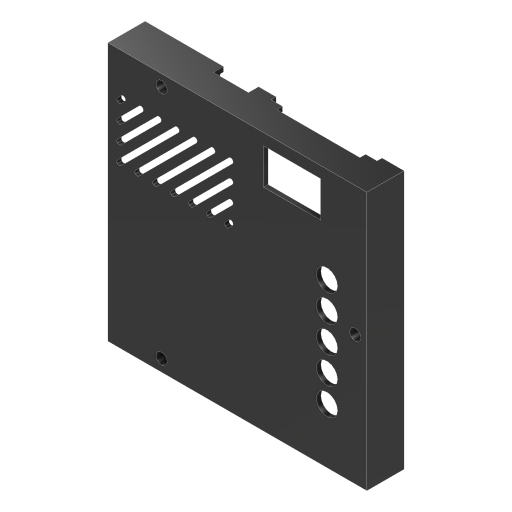
# Autodesk Inventor part: display_cover_part1_back
Saved by Autodesk Inventor 2023 (Build 270158000, 158)
## iProperties
Created: 2024-12-14
Part Number: display_cover_part1_back
Material: Všeobecné
Document SubType Name: Modeling
Designer: Marek
Density: 1 g/cm^3
Appearance: Lesklá – černá
Author: Marek
## iProperties of the stored document display_cover_part1_back_3D tisk.ipt
Created: 2025-02-02
Part Number: display_cover_part1_back_3D tisk
Material: Všeobecné
Document SubType Name: Modeling
Designer: Marek
Density: 1 g/cm^3
Appearance: Výchozí
Author: Marek
Autodesk Inventor part; units mm, degrees
ref_plane "YZ Plane" through (0, 0, 0) normal (1, 0, 0) x (0, 1, 0)
ref_plane "XZ Plane" through (0, 0, 0) normal (0, 1, 0) x (-1, 0, 0)
ref_plane "XY Plane" through (0, 0, 0) normal (0, 0, 1) x (1, 0, 0)
sketch "Náčrt1" plane through (0, 0, 0) normal (0, 0, 1) x (1, 0, 0)
  line L0 (0, 110.95) -> (0, -110.95) projected
  line L1 (-107, 0) -> (115.25, 0) projected
  line L2 (-75.25, 79.25) -> (83.5, 79.25)
  line L3 (83.5, 79.25) -> (83.5, -79.25)
  line L4 (83.5, -79.25) -> (-75.25, -79.25)
  line L5 (-75.25, -79.25) -> (-75.25, 79.25)
  point P0 (0, 0)
  dimension "d0" = 158.75
  dimension "d1" = 158.5
  dimension "d7" = 83.5
  constraints: 8 end point, 2 parallel, 1 horizontal, 1 perpendicular, 1 other
  measures "d0" distance of L3.end L4.end
  measures "d1" distance of L2.end L3.end
  measures "d7" distance between parallel lines of L0 L3
extrude "Vysunutí1" add sketch "Náčrt1" along normal blind 2.8
sketch "Náčrt2" plane through (0, 0, 0) normal (0, 0, -1) x (-1, 0, 0)
  line L0 (75.25, -79.25) -> (-83.5, -79.25) projected
  line L1 (75.25, 79.25) -> (75.25, -79.25) projected
  line L2 (-83.5, 79.25) -> (75.25, 79.25) projected
  line L3 (-83.5, -79.25) -> (-83.5, 79.25) projected
  line L4 (-115.3, 0) -> (107.3, 0) projected
  line L5 (0, -110.95) -> (0, 110.95) projected
  line L6 (-83.5, -79.25) -> (-83.5, 79.25) projected
  line L7 (75.25, 79.25) -> (75.25, -79.25) projected
  line L8 (-83.5, 79.25) -> (75.25, 79.25)
  line L9 (75.25, 79.25) -> (75.25, -79.25)
  line L10 (75.25, -79.25) -> (-83.5, -79.25)
  line L11 (-83.5, -79.25) -> (-83.5, 79.25)
  line L12 (-79.5, 76.25) -> (75.25, 76.25)
  line L13 (75.25, -75.25) -> (-79.5, -75.25)
  line L14 (-79.5, -75.25) -> (-79.5, 76.25)
  arc A0 (-79.5, -13.6771) -> (-79.5, 13.6771) centre (-83.5, 0) ccw
  line L15 (-83.5, 79.25) -> (75.25, 79.25) projected
  arc A1 (28.4194, 76.25) -> (56.2806, 76.25) centre (42.35, 79.25) ccw
  line L16 (75.25, -79.25) -> (-83.5, -79.25) projected
  arc A2 (56.0271, -75.25) -> (28.6729, -75.25) centre (42.35, -79.25) ccw
  line L17 (75.25, 79.25) -> (75.25, 76.25)
  line L18 (75.25, -75.25) -> (75.25, -79.25)
  point P0 (0, 0)
  point P1 (75.25, 76.25)
  point P2 (75.25, -75.25)
  dimension "d4" = 3
  dimension "d5" = 4
  dimension "d6" = 4
  dimension "d8" = 28.5
  dimension "d9" = 28.5
  dimension "d10" = 42.35
  dimension "d12" = 42.35
  dimension "d13" = 14.25
  constraints: 18 end point, 10 point on line, 6 point on circle, 3 centre point, 3 parallel, 3 perpendicular, 2 collinear, 2 horizontal, 1 midpoint
  measures "d4" distance between parallel lines of L2 L12
  measures "d5" distance between parallel lines of L14 L3
  measures "d6" distance between parallel lines of L13 L10
  measures "d8" diameter of A0
  measures "d9" diameter of A1
  measures "d10" distance from line of A1.centre L5
  measures "d12" distance from line of L5 A2.centre
  measures "d13" radius of A2
extrude "Vysunutí2" add sketch "Náčrt2" along normal blind 20 contours L0 L5 L13 L1 | L0 L3 L4 L14 L13 L5 | L13 A2 | L3 L2 L5 L12 L14 L4 | L12 L5 L2 L1 | L14 A0 L4 | L4 A0 L14 | A1 L12
sketch "Náčrt3" plane through (0, 0, -20) normal (0, 0, -1) x (-1, 0, 0)
  arc A0 (28.4194, 76.25) -> (56.2806, 76.25) centre (42.35, 79.25) ccw projected
  line L0 (56.2806, 76.25) -> (75.25, 76.25) projected
  line L1 (75.25, 76.25) -> (75.25, 79.25) projected
  line L2 (75.25, 79.25) -> (-83.5, 79.25) projected
  line L3 (-83.5, 79.25) -> (-83.5, -79.25) projected
  line L4 (-83.5, -79.25) -> (75.25, -79.25) projected
  line L5 (75.25, -79.25) -> (75.25, -75.25) projected
  line L6 (75.25, -75.25) -> (56.0271, -75.25) projected
  arc A1 (56.0271, -75.25) -> (28.6729, -75.25) centre (42.35, -79.25) ccw projected
  line L7 (28.6729, -75.25) -> (-79.5, -75.25) projected
  line L8 (-79.5, -75.25) -> (-79.5, -13.6771) projected
  arc A2 (-79.5, -13.6771) -> (-79.5, 13.6771) centre (-83.5, 0) ccw projected
  line L9 (-79.5, 13.6771) -> (-79.5, 76.25) projected
  line L10 (-79.5, 76.25) -> (28.4194, 76.25) projected
  arc A3 (-79.5, -13.6771) -> (-79.5, 13.6771) centre (-83.5, 0) ccw projected
  circle A4 centre (42.35, 79.25) radius 14.25
  circle A5 centre (-83.5, 0) radius 14.25
  arc A6 (56.0271, -75.25) -> (28.6729, -75.25) centre (42.35, -79.25) ccw projected
  circle A7 centre (42.35, -79.25) radius 14.25
  line L11 (33.6036, 68) -> (51.0964, 68)
  line L12 (33.6036, -68) -> (51.0964, -68)
  line L13 (-72.25, 8.7464) -> (-72.25, -8.7464)
  point P0 (0, 0)
  point P1 (42.35, 65)
  point P2 (42.35, -65)
  point P3 (-69.25, 0)
  dimension "d16" = 3
  dimension "d17" = 3
  dimension "d18" = 3
  constraints: 11 point on circle, 6 end point, 3 centre point, 3 coincident, 2 horizontal, 1 concentric, 1 vertical
  measures "d16" distance from line of L11 point (42.35, 65)
  measures "d17" distance from line of point (42.35, -65) L12
  measures "d18" distance from line of point (-69.25, 0) L13
extrude "Vysunutí3" cut sketch "Náčrt3" against normal blind 4 contours L11 A0 | A2 L13 | A1 L12
sketch "Náčrt4" plane through (0, 0, 2.8) normal (0, 0, 1) x (1, 0, 0)
  line L0 (0, 110.95) -> (0, -110.95) projected
  line L1 (-107.3, 0) -> (115.3, 0) projected
  line L2 (-75.25, -79.25) -> (83.5, -79.25) projected
  line L3 (83.5, -79.25) -> (83.5, 79.25) projected
  line L4 (83.5, 79.25) -> (-75.25, 79.25) projected
  line L5 (-75.25, 79.25) -> (-75.25, -79.25) projected
  line L6 (-36.416, 17.834) -> (1.0607, 55.3107) construction
  line L7 (-36.416, 19.9553) -> (-1.0607, 55.3107)
  line L8 (1.0607, 53.1893) -> (-34.2947, 17.834)
  arc A0 (-36.416, 19.9553) -> (-34.2947, 17.834) centre (-35.3553, 18.8947) ccw
  arc A1 (1.0607, 53.1893) -> (-1.0607, 55.3107) centre (0, 54.25) ccw
  arc A2 (-47.416, 19.9553) -> (-45.2947, 17.834) centre (-46.3553, 18.8947) ccw
  line L9 (-47.416, 19.9553) -> (-12.0607, 55.3107)
  line L10 (-47.416, 17.834) -> (-9.9393, 55.3107) construction
  line L11 (-9.9393, 53.1893) -> (-45.2947, 17.834)
  arc A3 (-9.9393, 53.1893) -> (-12.0607, 55.3107) centre (-11, 54.25) ccw
  arc A4 (-58.416, 19.9553) -> (-56.2947, 17.834) centre (-57.3553, 18.8947) ccw
  line L12 (-58.416, 19.9553) -> (-23.0607, 55.3107)
  line L13 (-58.416, 17.834) -> (-20.9393, 55.3107) construction
  line L14 (-20.9393, 53.1893) -> (-56.2947, 17.834)
  arc A5 (-20.9393, 53.1893) -> (-23.0607, 55.3107) centre (-22, 54.25) ccw
  arc A6 (-69.416, 19.9553) -> (-67.2947, 17.834) centre (-68.3553, 18.8947) ccw
  line L15 (-69.416, 19.9553) -> (-34.0607, 55.3107)
  line L16 (-69.416, 17.834) -> (-31.9393, 55.3107) construction
  line L17 (-31.9393, 53.1893) -> (-67.2947, 17.834)
  arc A7 (-31.9393, 53.1893) -> (-34.0607, 55.3107) centre (-33, 54.25) ccw
  line L18 (-25.416, 17.834) -> (1.0607, 44.3107) construction
  line L19 (-25.416, 19.9553) -> (-1.0607, 44.3107)
  line L20 (1.0607, 42.1893) -> (-23.2947, 17.834)
  arc A8 (-25.416, 19.9553) -> (-23.2947, 17.834) centre (-24.3553, 18.8947) ccw
  arc A9 (1.0607, 42.1893) -> (-1.0607, 44.3107) centre (0, 43.25) ccw
  line L21 (-14.416, 17.834) -> (1.0607, 33.3107) construction
  line L22 (-14.416, 19.9553) -> (-1.0607, 33.3107)
  line L23 (1.0607, 31.1893) -> (-12.2947, 17.834)
  arc A10 (-14.416, 19.9553) -> (-12.2947, 17.834) centre (-13.3553, 18.8947) ccw
  arc A11 (1.0607, 31.1893) -> (-1.0607, 33.3107) centre (0, 32.25) ccw
  line L24 (-52.1324, 18.6176) -> (-15.5772, 55.1728) construction
  line L25 (-69.416, 28.834) -> (-42.9393, 55.3107) construction
  line L26 (-67.2947, 28.834) -> (-42.9393, 53.1893)
  line L27 (-45.0607, 55.3107) -> (-69.416, 30.9553)
  arc A12 (-69.416, 30.9553) -> (-67.2947, 28.834) centre (-68.3553, 29.8947) ccw
  arc A13 (-42.9393, 53.1893) -> (-45.0607, 55.3107) centre (-44, 54.25) ccw
  line L28 (-69.416, 39.834) -> (-53.9393, 55.3107) construction
  line L29 (-69.416, 41.9553) -> (-56.0607, 55.3107)
  line L30 (-53.9393, 53.1893) -> (-67.2947, 39.834)
  arc A14 (-69.416, 41.9553) -> (-67.2947, 39.834) centre (-68.3553, 40.8947) ccw
  arc A15 (-53.9393, 53.1893) -> (-56.0607, 55.3107) centre (-55, 54.25) ccw
  line L31 (-68.3553, 18.8947) -> (-68.3553, 54.25) construction
  line L32 (0, 54.25) -> (-68.3553, 54.25) construction
  line L33 (-3.416, 17.834) -> (1.0607, 22.3107) construction
  line L34 (-1.2947, 17.834) -> (1.0607, 20.1893)
  line L35 (-1.0607, 22.3107) -> (-3.416, 19.9553)
  arc A16 (-3.416, 19.9553) -> (-1.2947, 17.834) centre (-2.3553, 18.8947) ccw
  arc A17 (1.0607, 20.1893) -> (-1.0607, 22.3107) centre (0, 21.25) ccw
  line L36 (-69.416, 50.834) -> (-64.9393, 55.3107) construction
  line L37 (-67.2947, 50.834) -> (-64.9393, 53.1893)
  line L38 (-67.0607, 55.3107) -> (-69.416, 52.9553)
  arc A18 (-69.416, 52.9553) -> (-67.2947, 50.834) centre (-68.3553, 51.8947) ccw
  arc A19 (-64.9393, 53.1893) -> (-67.0607, 55.3107) centre (-66, 54.25) ccw
  point P0 (0, 0)
  point P1 (-17.6777, 36.5723)
  point P2 (-28.6777, 36.5723)
  point P3 (-39.6777, 36.5723)
  point P4 (-50.6777, 36.5723)
  point P5 (-12.1777, 31.0723)
  point P6 (-6.6777, 25.5723)
  point P7 (-56.1777, 42.0723)
  point P8 (-61.6777, 47.5723)
  point P9 (-1.1777, 20.0723)
  point P10 (-67.1777, 53.0723)
  dimension "d21" = 45
  dimension "d22" = 50
  dimension "d23" = 3
  dimension "d24" = 25
  dimension "d27" = 11
  dimension "d32" = 3
  dimension "d33" = 45
  dimension "d36" = 11
  dimension "d38" = 3
  dimension "d39" = 45
  dimension "d40" = 11
  dimension "d42" = 11
  dimension "d43" = 11
  dimension "d44" = 11
  dimension "d45" = 11
  dimension "d46" = 11
  dimension "d47" = 11
  dimension "d48" = 3
  dimension "d49" = 3
  dimension "d52" = 3
  dimension "d53" = 45
  dimension "d54" = 11
  dimension "d55" = 11
  dimension "d56" = 3
  dimension "d57" = 11
  dimension "d58" = 11
  constraints: 86 end point, 60 point on circle, 29 point on line, 28 tangent, 20 centre point, 9 parallel, 7 midpoint, 1 horizontal, 1 perpendicular, 43 other
  measures "d21" angle of L1 L6
  measures "d22" distance of A0.centre L32.start
  measures "d23" distance between parallel lines of L8 L7
  measures "d24" distance from line of L4 L32.start
  measures "d27" distance of L7.start L9.start
  measures "d32" distance between parallel lines of L20 L19
  measures "d33" angle of L18 L1
  measures "d36" distance of A0.centre A8.centre
  measures "d38" distance between parallel lines of L23 L22
  measures "d39" angle of L1 L21
  measures "d40" distance of A8.centre A10.centre
  measures "d42" distance of A9.centre A11.centre
  measures "d43" distance of A9.centre L32.start
  measures "d44" distance of A7.centre A13.centre
  measures "d45" distance of A13.centre A15.centre
  measures "d46" distance of L31.start A12.centre
  measures "d47" distance of A12.centre A14.centre
  measures "d48" distance between parallel lines of L27 L26
  measures "d49" distance between parallel lines of L29 L30
  measures "d52" diameter of A17
  measures "d53" angle of L1 L33
  measures "d54" distance of A10.centre A16.centre
  measures "d55" distance of A17.centre A11.centre
  measures "d56" distance between parallel lines of L38 L37
  measures "d57" distance of A15.centre A19.centre
  measures "d58" distance of A14.centre A18.centre
extrude "Vysunutí4" cut sketch "Náčrt4" against normal through all contours A1 L8 L0 | L0 L8 A0 L7 A1 | A9 L20 L0 | L0 L20 A8 L19 A9 | L34 A16 L35 A17 L0 | L0 A17 L34 | A11 L23 L0 | L0 L23 A10 L22 A11 | L9 A3 L11 A2 | L12 A5 L14 A4 | L15 A7 L17 A6 | A12 L27 A13 L26 | L29 A15 L30 A14 | A18 L38 A19 L37
sketch "Náčrt5" plane through (-75.25, 79.25, 2.8) normal (0, 1, 0) x (1, 0, 0)
  line L0 (0, 22.8) -> (0, 0) projected
  line L1 (158.75, 0) -> (0, 0) projected
  line L2 (158.75, 22.8) -> (158.75, 0) projected
  line L3 (0, 22.8) -> (158.75, 22.8) projected
  line L4 (75.25, 27.36) -> (75.25, -4.56) projected
  line L5 (190.8, 2.8) -> (-31.8, 2.8) projected
  line L6 (158.75, 22.8) -> (0, 22.8) projected
  line L7 (80.25, 22.8) -> (145.25, 22.8)
  line L8 (145.25, 22.8) -> (145.25, 16.25)
  line L9 (145.25, 16.25) -> (80.25, 16.25)
  line L10 (80.25, 16.25) -> (80.25, 22.8)
  line L11 (145.25, 16.25) -> (138.25, 16.25)
  line L12 (138.25, 16.25) -> (138.25, 19.75)
  line L13 (138.25, 19.75) -> (145.25, 19.75)
  line L14 (145.25, 19.75) -> (145.25, 16.25)
  line L15 (80.25, 16.25) -> (87.25, 16.25)
  line L16 (87.25, 16.25) -> (87.25, 19.75)
  line L17 (87.25, 19.75) -> (80.25, 19.75)
  line L18 (80.25, 19.75) -> (80.25, 16.25)
  point P0 (75.25, 2.8)
  dimension "d59" = 6.55
  dimension "d60" = 65
  dimension "d61" = 13.5
  dimension "d62" = 7
  dimension "d63" = 3.5
  dimension "d64" = 7
  dimension "d65" = 3.5
  constraints: 24 end point, 6 parallel, 3 horizontal, 3 perpendicular, 1 point on line
  measures "d59" distance of L7.end L8.end
  measures "d60" distance between parallel lines of L8 L10
  measures "d61" distance between parallel lines of L2 L8
  measures "d62" distance of L12.end L13.end
  measures "d63" distance of L11.end L12.end
  measures "d64" distance of L17.end L16.end
  measures "d65" distance of L16.end L15.end
extrude "Vysunutí5" cut sketch "Náčrt5" against normal up to surface (3 mm away) contours L3 L8 L13 L12 L9 L16 L17 L10
sketch "Náčrt6" plane through (-75.25, 79.25, 2.8) normal (0, 1, 0) x (1, 0, 0)
  line L0 (145.25, 22.8) -> (145.25, 19.75) projected
  line L1 (145.25, 19.75) -> (138.25, 19.75) projected
  line L2 (138.25, 19.75) -> (138.25, 16.25) projected
  line L3 (138.25, 16.25) -> (87.25, 16.25) projected
  line L4 (87.25, 16.25) -> (87.25, 19.75) projected
  line L5 (87.25, 19.75) -> (80.25, 19.75) projected
  line L6 (80.25, 19.75) -> (80.25, 22.8) projected
  line L7 (0, 22.8) -> (80.25, 22.8) projected
  line L8 (0, 22.8) -> (0, 0) projected
  line L9 (158.75, 0) -> (0, 0) projected
  line L10 (158.75, 22.8) -> (158.75, 0) projected
  line L11 (145.25, 22.8) -> (158.75, 22.8) projected
  line L12 (158.75, 22.8) -> (0, 22.8) projected
  line L13 (47.96, 22.8) -> (67.26, 22.8)
  line L14 (67.26, 22.8) -> (67.26, 16.6)
  line L15 (67.26, 16.6) -> (47.96, 16.6)
  line L16 (47.96, 16.6) -> (47.96, 22.8)
  point P0 (75.25, 2.8)
  dimension "d68" = 91.49
  dimension "d69" = 19.3
  dimension "d70" = 6.2
  constraints: 8 end point, 2 parallel, 1 horizontal, 1 perpendicular, 1 point on line
  measures "d68" distance between parallel lines of L10 L14
  measures "d69" distance between parallel lines of L16 L14
  measures "d70" distance between parallel lines of L13 L15
extrude "Vysunutí6" cut sketch "Náčrt6" against normal up to surface (3 mm away) contours L14 L15 L16 L7
sketch "Náčrt7" plane through (0, 0, 2.8) normal (0, 0, 1) x (1, 0, 0)
  arc A0 (-69.416, 41.9553) -> (-67.2947, 39.834) centre (-68.3553, 40.8947) ccw projected
  line L0 (-69.416, 41.9553) -> (-56.0607, 55.3107) projected
  arc A1 (-53.9393, 53.1893) -> (-56.0607, 55.3107) centre (-55, 54.25) ccw projected
  line L1 (-53.9393, 53.1893) -> (-67.2947, 39.834) projected
  arc A2 (-47.416, 19.9553) -> (-45.2947, 17.834) centre (-46.3553, 18.8947) ccw projected
  line L2 (-47.416, 19.9553) -> (-12.0607, 55.3107) projected
  arc A3 (-9.9393, 53.1893) -> (-12.0607, 55.3107) centre (-11, 54.25) ccw projected
  line L3 (-9.9393, 53.1893) -> (-45.2947, 17.834) projected
  arc A4 (1.0607, 31.1893) -> (-1.0607, 33.3107) centre (0, 32.25) ccw projected
  line L4 (1.0607, 31.1893) -> (-12.2947, 17.834) projected
  arc A5 (-14.416, 19.9553) -> (-12.2947, 17.834) centre (-13.3553, 18.8947) ccw projected
  line L5 (-14.416, 19.9553) -> (-1.0607, 33.3107) projected
  arc A6 (-58.416, 19.9553) -> (-56.2947, 17.834) centre (-57.3553, 18.8947) ccw projected
  line L6 (-58.416, 19.9553) -> (-23.0607, 55.3107) projected
  arc A7 (-20.9393, 53.1893) -> (-23.0607, 55.3107) centre (-22, 54.25) ccw projected
  line L7 (-20.9393, 53.1893) -> (-56.2947, 17.834) projected
  arc A8 (1.0607, 20.1893) -> (-1.0607, 22.3107) centre (0, 21.25) ccw projected
  line L8 (1.0607, 20.1893) -> (-1.2947, 17.834) projected
  arc A9 (-3.416, 19.9553) -> (-1.2947, 17.834) centre (-2.3553, 18.8947) ccw projected
  line L9 (-3.416, 19.9553) -> (-1.0607, 22.3107) projected
  line L10 (-69.416, 30.9553) -> (-45.0607, 55.3107) projected
  arc A10 (-42.9393, 53.1893) -> (-45.0607, 55.3107) centre (-44, 54.25) ccw projected
  line L11 (-42.9393, 53.1893) -> (-67.2947, 28.834) projected
  arc A11 (-69.416, 30.9553) -> (-67.2947, 28.834) centre (-68.3553, 29.8947) ccw projected
  arc A12 (1.0607, 53.1893) -> (-1.0607, 55.3107) centre (0, 54.25) ccw projected
  line L12 (1.0607, 53.1893) -> (-34.2947, 17.834) projected
  arc A13 (-36.416, 19.9553) -> (-34.2947, 17.834) centre (-35.3553, 18.8947) ccw projected
  line L13 (-36.416, 19.9553) -> (-1.0607, 55.3107) projected
  arc A14 (1.0607, 42.1893) -> (-1.0607, 44.3107) centre (0, 43.25) ccw projected
  line L14 (1.0607, 42.1893) -> (-23.2947, 17.834) projected
  arc A15 (-25.416, 19.9553) -> (-23.2947, 17.834) centre (-24.3553, 18.8947) ccw projected
  line L15 (-25.416, 19.9553) -> (-1.0607, 44.3107) projected
  arc A16 (-69.416, 19.9553) -> (-67.2947, 17.834) centre (-68.3553, 18.8947) ccw projected
  line L16 (-69.416, 19.9553) -> (-34.0607, 55.3107) projected
  arc A17 (-31.9393, 53.1893) -> (-34.0607, 55.3107) centre (-33, 54.25) ccw projected
  line L17 (-31.9393, 53.1893) -> (-67.2947, 17.834) projected
  line L18 (-69.416, 52.9553) -> (-67.0607, 55.3107) projected
  arc A18 (-64.9393, 53.1893) -> (-67.0607, 55.3107) centre (-66, 54.25) ccw projected
  line L19 (-64.9393, 53.1893) -> (-67.2947, 50.834) projected
  arc A19 (-69.416, 52.9553) -> (-67.2947, 50.834) centre (-68.3553, 51.8947) ccw projected
  line L20 (-75.25, -79.25) -> (83.5, -79.25) projected
  line L21 (83.5, -79.25) -> (83.5, 79.25) projected
  line L22 (83.5, 79.25) -> (-75.25, 79.25) projected
  line L23 (-75.25, 79.25) -> (-75.25, -79.25) projected
  arc A20 (-56.2806, 76.25) -> (-28.4194, 76.25) centre (-42.35, 79.25) ccw projected
  arc A21 (79.5, 13.6771) -> (79.5, -13.6771) centre (83.5, 0) ccw projected
  arc A22 (-28.6729, -75.25) -> (-56.0271, -75.25) centre (-42.35, -79.25) ccw projected
  line L24 (0, 110.95) -> (0, -110.95) projected
  line L25 (-107, 0) -> (115.25, 0) projected
  point P0 (0, 0)
  point P1 (-42.35, 72.125)
  point P2 (76.375, 0)
  point P3 (-42.35, -72.125)
  dimension "d73" = 7.125
  dimension "d74" = 7.125
  dimension "d75" = 7.125
  dimension "d76" = 42.35
  dimension "d77" = 42.35
  constraints: 1 point on line
  measures "d73" distance from line of L22 point (-42.35, 72.125)
  measures "d74" distance from line of point (76.375, 0) L21
  measures "d75" distance from line of L20 point (-42.35, -72.125)
  measures "d76" distance from line of L24 point (-42.35, 72.125)
  measures "d77" distance from line of L24 point (-42.35, -72.125)
hole "Díra1" at (-42.35, 72.125, 2.8) at (76.375, 0, 2.8) at (-42.35, -72.125, 2.8) direction (0, 0, -1) diameter 7 depth 6
sketch "Náčrt8" plane through (-42.35, 72.125, -3.2) normal (0, 0, 1) x (1, 0, 0)
  circle A0 centre (0, 0) radius 3.5 projected
  circle A1 centre (0, -144.25) radius 3.5 projected
  circle A2 centre (118.725, -72.125) radius 3.5 projected
  point P0 (42.35, -72.125)
  constraints: 3 coincident
hole "Díra2" at (-42.35, 72.125, -3.2) at (76.375, 0, -3.2) at (-42.35, -72.125, -3.2) direction (0, 0, -1) diameter 3.4 depth 16.8
sketch "Náčrt9" plane through (0, 0, 2.8) normal (0, 0, 1) x (1, 0, 0)
  circle A0 centre (76.375, 0) radius 3.5 projected
  circle A1 centre (-42.35, 72.125) radius 3.5 projected
  circle A2 centre (-42.35, -72.125) radius 3.5 projected
  arc A3 (-69.416, 41.9553) -> (-67.2947, 39.834) centre (-68.3553, 40.8947) ccw projected
  line L0 (-69.416, 41.9553) -> (-56.0607, 55.3107) projected
  arc A4 (-53.9393, 53.1893) -> (-56.0607, 55.3107) centre (-55, 54.25) ccw projected
  line L1 (-53.9393, 53.1893) -> (-67.2947, 39.834) projected
  arc A5 (-47.416, 19.9553) -> (-45.2947, 17.834) centre (-46.3553, 18.8947) ccw projected
  line L2 (-47.416, 19.9553) -> (-12.0607, 55.3107) projected
  arc A6 (-9.9393, 53.1893) -> (-12.0607, 55.3107) centre (-11, 54.25) ccw projected
  line L3 (-9.9393, 53.1893) -> (-45.2947, 17.834) projected
  arc A7 (1.0607, 31.1893) -> (-1.0607, 33.3107) centre (0, 32.25) ccw projected
  line L4 (1.0607, 31.1893) -> (-12.2947, 17.834) projected
  arc A8 (-14.416, 19.9553) -> (-12.2947, 17.834) centre (-13.3553, 18.8947) ccw projected
  line L5 (-14.416, 19.9553) -> (-1.0607, 33.3107) projected
  arc A9 (-58.416, 19.9553) -> (-56.2947, 17.834) centre (-57.3553, 18.8947) ccw projected
  line L6 (-58.416, 19.9553) -> (-23.0607, 55.3107) projected
  arc A10 (-20.9393, 53.1893) -> (-23.0607, 55.3107) centre (-22, 54.25) ccw projected
  line L7 (-20.9393, 53.1893) -> (-56.2947, 17.834) projected
  arc A11 (1.0607, 20.1893) -> (-1.0607, 22.3107) centre (0, 21.25) ccw projected
  line L8 (1.0607, 20.1893) -> (-1.2947, 17.834) projected
  arc A12 (-3.416, 19.9553) -> (-1.2947, 17.834) centre (-2.3553, 18.8947) ccw projected
  line L9 (-3.416, 19.9553) -> (-1.0607, 22.3107) projected
  line L10 (-69.416, 30.9553) -> (-45.0607, 55.3107) projected
  arc A13 (-42.9393, 53.1893) -> (-45.0607, 55.3107) centre (-44, 54.25) ccw projected
  line L11 (-42.9393, 53.1893) -> (-67.2947, 28.834) projected
  arc A14 (-69.416, 30.9553) -> (-67.2947, 28.834) centre (-68.3553, 29.8947) ccw projected
  arc A15 (1.0607, 53.1893) -> (-1.0607, 55.3107) centre (0, 54.25) ccw projected
  line L12 (1.0607, 53.1893) -> (-34.2947, 17.834) projected
  arc A16 (-36.416, 19.9553) -> (-34.2947, 17.834) centre (-35.3553, 18.8947) ccw projected
  line L13 (-36.416, 19.9553) -> (-1.0607, 55.3107) projected
  arc A17 (1.0607, 42.1893) -> (-1.0607, 44.3107) centre (0, 43.25) ccw projected
  line L14 (1.0607, 42.1893) -> (-23.2947, 17.834) projected
  arc A18 (-25.416, 19.9553) -> (-23.2947, 17.834) centre (-24.3553, 18.8947) ccw projected
  line L15 (-25.416, 19.9553) -> (-1.0607, 44.3107) projected
  arc A19 (-69.416, 19.9553) -> (-67.2947, 17.834) centre (-68.3553, 18.8947) ccw projected
  line L16 (-69.416, 19.9553) -> (-34.0607, 55.3107) projected
  arc A20 (-31.9393, 53.1893) -> (-34.0607, 55.3107) centre (-33, 54.25) ccw projected
  line L17 (-31.9393, 53.1893) -> (-67.2947, 17.834) projected
  line L18 (-69.416, 52.9553) -> (-67.0607, 55.3107) projected
  arc A21 (-64.9393, 53.1893) -> (-67.0607, 55.3107) centre (-66, 54.25) ccw projected
  line L19 (-64.9393, 53.1893) -> (-67.2947, 50.834) projected
  arc A22 (-69.416, 52.9553) -> (-67.2947, 50.834) centre (-68.3553, 51.8947) ccw projected
  line L20 (-75.25, -79.25) -> (83.5, -79.25) projected
  line L21 (83.5, -79.25) -> (83.5, 79.25) projected
  line L22 (83.5, 79.25) -> (-75.25, 79.25) projected
  line L23 (-75.25, 79.25) -> (-75.25, -79.25) projected
  line L24 (-107, 0) -> (115.25, 0) projected
  line L25 (0, 110.95) -> (0, -110.95) projected
  line L26 (20.15, 72.25) -> (55.15, 72.25)
  line L27 (55.15, 72.25) -> (55.15, 50.25)
  line L28 (55.15, 50.25) -> (20.15, 50.25)
  line L29 (20.15, 50.25) -> (20.15, 72.25)
  point P0 (0, 0)
  point P1 (37.65, 72.25)
  dimension "d92" = 45.85
  dimension "d93" = 7
  dimension "d94" = 22
  dimension "d95" = 35
  constraints: 8 end point, 2 parallel, 1 horizontal, 1 midpoint, 1 perpendicular
  measures "d92" distance from line of L21 point (37.65, 72.25)
  measures "d93" distance between parallel lines of L22 L26
  measures "d94" distance between parallel lines of L26 L28
  measures "d95" distance between parallel lines of L29 L27
extrude "Vysunutí7" cut sketch "Náčrt9" against normal up to surface (2.8 mm away) contours L26 L27 L28 L29
sketch "Náčrt10" plane through (0, 0, 2.8) normal (0, 0, 1) x (1, 0, 0)
  line L0 (55.15, 50.25) -> (20.15, 50.25) projected
  line L1 (20.15, 50.25) -> (20.15, 72.25) projected
  line L2 (20.15, 72.25) -> (55.15, 72.25) projected
  line L3 (55.15, 72.25) -> (55.15, 50.25) projected
  circle A0 centre (76.375, 0) radius 3.5 projected
  circle A1 centre (-42.35, 72.125) radius 3.5 projected
  circle A2 centre (-42.35, -72.125) radius 3.5 projected
  arc A3 (-69.416, 41.9553) -> (-67.2947, 39.834) centre (-68.3553, 40.8947) ccw projected
  line L4 (-69.416, 41.9553) -> (-56.0607, 55.3107) projected
  arc A4 (-53.9393, 53.1893) -> (-56.0607, 55.3107) centre (-55, 54.25) ccw projected
  line L5 (-53.9393, 53.1893) -> (-67.2947, 39.834) projected
  arc A5 (-47.416, 19.9553) -> (-45.2947, 17.834) centre (-46.3553, 18.8947) ccw projected
  line L6 (-47.416, 19.9553) -> (-12.0607, 55.3107) projected
  arc A6 (-9.9393, 53.1893) -> (-12.0607, 55.3107) centre (-11, 54.25) ccw projected
  line L7 (-9.9393, 53.1893) -> (-45.2947, 17.834) projected
  arc A7 (1.0607, 31.1893) -> (-1.0607, 33.3107) centre (0, 32.25) ccw projected
  line L8 (1.0607, 31.1893) -> (-12.2947, 17.834) projected
  arc A8 (-14.416, 19.9553) -> (-12.2947, 17.834) centre (-13.3553, 18.8947) ccw projected
  line L9 (-14.416, 19.9553) -> (-1.0607, 33.3107) projected
  arc A9 (-58.416, 19.9553) -> (-56.2947, 17.834) centre (-57.3553, 18.8947) ccw projected
  line L10 (-58.416, 19.9553) -> (-23.0607, 55.3107) projected
  arc A10 (-20.9393, 53.1893) -> (-23.0607, 55.3107) centre (-22, 54.25) ccw projected
  line L11 (-20.9393, 53.1893) -> (-56.2947, 17.834) projected
  arc A11 (1.0607, 20.1893) -> (-1.0607, 22.3107) centre (0, 21.25) ccw projected
  line L12 (1.0607, 20.1893) -> (-1.2947, 17.834) projected
  arc A12 (-3.416, 19.9553) -> (-1.2947, 17.834) centre (-2.3553, 18.8947) ccw projected
  line L13 (-3.416, 19.9553) -> (-1.0607, 22.3107) projected
  line L14 (-69.416, 30.9553) -> (-45.0607, 55.3107) projected
  arc A13 (-42.9393, 53.1893) -> (-45.0607, 55.3107) centre (-44, 54.25) ccw projected
  line L15 (-42.9393, 53.1893) -> (-67.2947, 28.834) projected
  arc A14 (-69.416, 30.9553) -> (-67.2947, 28.834) centre (-68.3553, 29.8947) ccw projected
  arc A15 (1.0607, 53.1893) -> (-1.0607, 55.3107) centre (0, 54.25) ccw projected
  line L16 (1.0607, 53.1893) -> (-34.2947, 17.834) projected
  arc A16 (-36.416, 19.9553) -> (-34.2947, 17.834) centre (-35.3553, 18.8947) ccw projected
  line L17 (-36.416, 19.9553) -> (-1.0607, 55.3107) projected
  arc A17 (1.0607, 42.1893) -> (-1.0607, 44.3107) centre (0, 43.25) ccw projected
  line L18 (1.0607, 42.1893) -> (-23.2947, 17.834) projected
  arc A18 (-25.416, 19.9553) -> (-23.2947, 17.834) centre (-24.3553, 18.8947) ccw projected
  line L19 (-25.416, 19.9553) -> (-1.0607, 44.3107) projected
  arc A19 (-69.416, 19.9553) -> (-67.2947, 17.834) centre (-68.3553, 18.8947) ccw projected
  line L20 (-69.416, 19.9553) -> (-34.0607, 55.3107) projected
  arc A20 (-31.9393, 53.1893) -> (-34.0607, 55.3107) centre (-33, 54.25) ccw projected
  line L21 (-31.9393, 53.1893) -> (-67.2947, 17.834) projected
  line L22 (-69.416, 52.9553) -> (-67.0607, 55.3107) projected
  arc A21 (-64.9393, 53.1893) -> (-67.0607, 55.3107) centre (-66, 54.25) ccw projected
  line L23 (-64.9393, 53.1893) -> (-67.2947, 50.834) projected
  arc A22 (-69.416, 52.9553) -> (-67.2947, 50.834) centre (-68.3553, 51.8947) ccw projected
  line L24 (-75.25, -79.25) -> (83.5, -79.25) projected
  line L25 (83.5, -79.25) -> (83.5, 79.25) projected
  line L26 (83.5, 79.25) -> (-75.25, 79.25) projected
  line L27 (-75.25, 79.25) -> (-75.25, -79.25) projected
  line L28 (0, 110.95) -> (0, -110.95) projected
  line L29 (-107, 0) -> (115.25, 0) projected
  line L30 (59, 38.1441) -> (59, -63.4041) construction
  point P0 (0, 0)
  point P1 (59, 3.88)
  point P2 (59, -12.63)
  point P3 (59, 20.39)
  point P4 (59, -29.14)
  point P5 (59, -45.65)
  dimension "d99" = 24.5
  dimension "d100" = 33.6
  dimension "d101" = 16.51
  dimension "d102" = 16.51
  dimension "d103" = 16.51
  dimension "d104" = 16.51
  constraints: 4 point on line, 2 end point, 1 midpoint, 1 parallel, 1 vertical
  measures "d99" distance between parallel lines of L25 L30
  measures "d100" distance from line of L24 point (59, -45.65)
  measures "d101" distance of point (59, -29.14) point (59, -45.65)
  measures "d102" distance of point (59, -29.14) point (59, -12.63)
  measures "d103" distance of point (59, -12.63) point (59, 3.88)
  measures "d104" distance of point (59, 3.88) point (59, 20.39)
hole "Díra3" at (59, 3.88, 2.8) at (59, -12.63, 2.8) at (59, 20.39, 2.8) at (59, -29.14, 2.8) at (59, -45.65, 2.8) direction (0, 0, -1) diameter 13 depth 2.8
sketch "Náčrt11" plane through (-7.99, 79.25, -20) normal (-1, 0, 0) x (0, 0, 1)
  line L0 (0, -3) -> (6.2, -3)
  line L1 (6.2, -3) -> (6.2, 1)
  line L2 (6.2, 1) -> (0, 1)
  line L3 (0, 1) -> (0, -3)
  point P0 (20, -79.25)
  dimension "d112" = 6.2
  dimension "d113" = 4
  constraints: 8 end point, 2 parallel, 1 horizontal, 1 perpendicular
  measures "d112" distance of L2.end L1.end
  measures "d113" distance between parallel lines of L0 L2
extrude "Vysunutí8" cut sketch "Náčrt11" against normal blind 2.3
sketch "Náčrt12" plane through (0, 0, 0) normal (0, 0, -1) x (-1, 0, 0)
  line L0 (0, -110.95) -> (0, 110.95) projected
  line L1 (-115.25, 0) -> (107, 0) projected
  line L2 (0, -60) -> (70, -60)
  line L3 (70, -60) -> (70, 0)
  line L4 (70, 0) -> (0, 0)
  line L5 (0, 0) -> (0, -60)
  dimension "d116" = 60
  dimension "d117" = 70
  constraints: 8 end point, 2 parallel, 2 point on line, 1 horizontal, 1 perpendicular
  measures "d116" distance between parallel lines of L1 L2
  measures "d117" distance between parallel lines of L0 L3
extrude "Vysunutí9" cut sketch "Náčrt12" against normal blind 1.5
